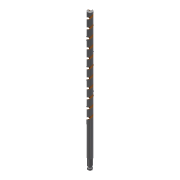
# Autodesk Inventor part: Auger bit
Saved by Autodesk Inventor 2014 SP1 (Build 180222100, 222)
## iProperties
Created: 2014-12-10
Part Number: Auger bit
Material: Generic
Document SubType Name: Modeling
Designer: AlecShufelt
Density: 1 g/cm^3
Appearance: Rust
Author: AlecShufelt
Autodesk Inventor part; units mm, degrees
ref_plane "YZ Plane" through (0, 0, 0) normal (1, 0, 0) x (0, 1, 0)
ref_plane "XZ Plane" through (0, 0, 0) normal (0, 1, 0) x (-1, 0, 0)
ref_plane "XY Plane" through (0, 0, 0) normal (0, 0, 1) x (1, 0, 0)
sketch "Sketch1" plane through (0, 0, 0) normal (0, 1, 0) x (-1, 0, 0)
  line L0 (-3.394877, -5.8801) -> (-6.789755, 0)
  line L1 (-6.789755, 0) -> (-3.394877, 5.8801)
  line L2 (-3.394877, 5.8801) -> (3.394877, 5.8801)
  line L3 (3.394877, 5.8801) -> (6.789755, 0)
  line L4 (6.789755, 0) -> (3.394877, -5.8801)
  line L5 (3.394877, -5.8801) -> (-3.394877, -5.8801)
  point P0 (0, 0)
  point P1 (0, 0)
  dimension "d0" = 11.7602
  constraints: 12 end point, 1 coincident, 13 other
  measures "d0" distance between parallel lines of L5 L2
extrude "Extrusion1" add sketch "Sketch1" along normal blind 5.334
sketch "Sketch2" plane through (0, 5.334, 0) normal (0, 1, 0) x (1, 0, 0)
  circle A0 centre (0, 0) radius 4.4196
  dimension "d3" = 8.8392
  constraints: 1 centre point, 1 coincident
  measures "d3" diameter of A0
extrude "Extrusion2" add sketch "Sketch2" along normal blind 4.5847
sketch "Sketch3" plane through (0, 9.9187, 0) normal (0, 1, 0) x (1, 0, 0)
  circle A0 centre (0, 0) radius 4.4196
  line L0 (-6.789755, 0) -> (-3.394877, 5.8801)
  line L1 (-3.394877, 5.8801) -> (3.394877, 5.8801)
  line L2 (3.394877, 5.8801) -> (6.789755, 0)
  line L3 (6.789755, 0) -> (3.394877, -5.8801)
  line L4 (3.394877, -5.8801) -> (-3.394877, -5.8801)
  line L5 (-3.394877, -5.8801) -> (-6.789755, 0)
  dimension "d6" = 11.7602
  constraints: 12 end point, 1 coincident, 13 other
  measures "d6" distance between parallel lines of L1 L4
extrude "Extrusion3" add sketch "Sketch3" along normal blind 22.606 contours A0 | L0 L1 L2 L3 L4 L5
fillet "Fillet1" radius 1.27 2 edges at (-4.4196, 9.9187, 0) (-4.4196, 5.334, 0)
sketch "Sketch4" plane through (0, 32.5247, 0) normal (0, 1, 0) x (1, 0, 0)
  circle A0 centre (0, 0) radius 7.9375
  dimension "d10" = 15.875
  constraints: 1 centre point, 1 coincident
  measures "d10" diameter of A0
extrude "Extrusion4" add sketch "Sketch4" along normal blind 406.4
sketch "Sketch5" plane through (0, 438.9247, 0) normal (0, 1, 0) x (1, 0, 0)
  circle A0 centre (0, 0) radius 7.9375 projected
  line L0 (0, 0) -> (0, 7.9375)
  line L1 (0, 0) -> (-7.9375, 0)
  constraints: 4 end point, 2 point on circle, 1 coincident, 1 perpendicular, 1 vertical
sketch "Sketch6" plane through (0, 0, 0) normal (1, 0, 0) x (0, 1, 0)
  line L0 (439.359168, 0) -> (425.628072, 0)
  line L1 (425.628072, 0) -> (450.13374, 0)
  point P0 (0, 0)
  constraints: 4 end point, 1 collinear, 1 horizontal
sketch "Sketch5 outline for Coil1" plane through (0, 438.9247, 0) normal (0, 1, 0) x (1, 0, 0)
  line L0 (-7.9375, 0) -> (0, 0)
  arc A0 (0, 7.9375) -> (-7.9375, 0) centre (0, 0) ccw
  line L1 (0, 0) -> (0, 7.9375)
coil "Coil1" sketch "Sketch5 outline for Coil1" operation cut axis through (0, 425.628072, 0) along (0, -1, 0) pitch 27.709091 turns 11 hand right
body "Solid1"
